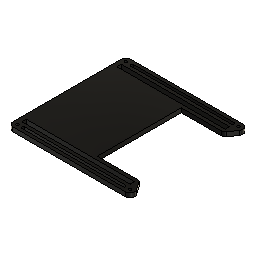
CameraBase v3 (Autodesk Fusion 360 design; units mm, degrees)
Autodesk Fusion 360 part; units mm, degrees
note: some values were not read from the file. Set by a fixed rule: which sketch regions a step uses.
sketch "Sketch1" plane through (0, 0, 0) normal (0, 0, 1) x (1, 0, 0)
  line L0 (-62.5, 60.2) -> (62.5, 60.2) construction
  line L1 (62.5, 60.2) -> (62.5, -60.2) construction
  line L2 (62.5, -60.2) -> (-62.5, -60.2) construction
  line L3 (-62.5, -60.2) -> (-62.5, 60.2) construction
  line L4 (0, 0) -> (0, 60.2) construction
  line L5 (0, 0) -> (-62.5, 0) construction
  circle A0 centre (62.5, 60.2) radius 1.5
  circle A1 centre (-62.5, 60.2) radius 1.5
  circle A2 centre (62.5, -60.2) radius 1.5
  circle A3 centre (-62.5, -60.2) radius 1.5
  line L6 (-62.5, -65.2) -> (62.5, -65.2)
  line L7 (-67.5, -60.2) -> (-67.5, 60.2)
  line L8 (-62.5, 65.2) -> (62.5, 65.2)
  line L9 (-56, 61.7) -> (56, 61.7)
  line L10 (-56, 58.7) -> (56, 58.7)
  arc A4 (-56, 61.7) -> (-56, 58.7) centre (-56, 60.2) ccw
  arc A5 (56, 58.7) -> (56, 61.7) centre (56, 60.2) ccw
  arc A6 (-67.5, 60.2) -> (-62.5, 65.2) centre (-62.5, 60.2) ccw construction
  arc A7 (-62.5, 65.2) -> (-67.5, 60.2) centre (-62.5, 60.2) ccw
  line L11 (-62.5, 55.2) -> (57.5, 55.2)
  line L12 (57.5, 55.2) -> (57.5, 50.4)
  line L13 (57.5, 50.4) -> (-62.5, 50.4)
  line L14 (-62.5, 50.4) -> (-62.5, 55.2)
  line L15 (66.6668, 57.4363) -> (60.6251, 48.3272)
  arc A8 (62.5, 65.2) -> (66.6668, 57.4363) centre (62.5, 60.2) ccw construction
  arc A9 (66.6668, 57.4363) -> (62.5, 65.2) centre (62.5, 60.2) ccw
  arc A10 (60.6251, 48.3272) -> (60.6251, 48.3272) centre (57.5, 50.4) ccw construction
  line L16 (-56, -58.7) -> (56, -58.7)
  line L17 (-56, -61.7) -> (56, -61.7)
  arc A11 (-56, -58.7) -> (-56, -61.7) centre (-56, -60.2) ccw
  arc A12 (56, -61.7) -> (56, -58.7) centre (56, -60.2) ccw
  line L18 (-62.5, -55.2) -> (57.5, -55.2)
  line L19 (57.5, -55.2) -> (57.5, -50.4)
  line L20 (57.5, -50.4) -> (-62.5, -50.4)
  line L21 (-62.5, -50.4) -> (-62.5, -55.2)
  line L22 (57.5, -60.2) -> (57.5, -55.2) construction
  line L23 (60.6251, -48.3272) -> (66.6668, -57.4363)
  line L24 (57.5, -46.65) -> (12.5, -46.65)
  line L25 (12.5, 46.65) -> (12.5, -46.65)
  arc A13 (57.5, -46.65) -> (60.6251, -48.3272) centre (57.5, -50.4) ccw construction
  arc A14 (60.6251, -48.3272) -> (57.5, -46.65) centre (57.5, -50.4) ccw
  arc A15 (66.6668, -57.4363) -> (62.5, -65.2) centre (62.5, -60.2) ccw construction
  arc A16 (62.5, -65.2) -> (66.6668, -57.4363) centre (62.5, -60.2) ccw
  arc A17 (-62.5, -65.2) -> (-67.5, -60.2) centre (-62.5, -60.2) ccw construction
  arc A18 (-67.5, -60.2) -> (-62.5, -65.2) centre (-62.5, -60.2) ccw
  line L26 (57.5, -50.4) -> (57.5, 50.4) construction
  line L27 (57.5, 46.65) -> (12.5, 46.65)
  arc A19 (60.6251, 48.3272) -> (57.5, 46.65) centre (57.5, 50.4) ccw construction
  arc A20 (57.5, 46.65) -> (60.6251, 48.3272) centre (57.5, 50.4) ccw
  line L28 (57.5, 55.2) -> (57.5, 60.2) construction
  point P0 (-62.5, 0)
  point P1 (0, 60.2)
  dimension "d1" = 125
  dimension "d2" = 120.4
  dimension "d3" = 3
  dimension "d4" = 3
  dimension "d5" = 3
  dimension "d6" = 3
  dimension "d7" = 10
  dimension "d8" = 10
  dimension "d9" = 10
  dimension "d10" = 10
  dimension "d11" = 3
  dimension "d12" = 5
  dimension "d13" = 6.5
  dimension "d14" = 6.5
  dimension "d16" = 4.8
  dimension "d17" = 5
  dimension "d19" = 3
  dimension "d20" = 5
  dimension "d21" = 6.5
  dimension "d22" = 6.5
  dimension "d23" = 4.8
  dimension "d24" = 7.5
  dimension "d25" = 50
  dimension "d28" = 3.75
  constraint horizontal L0
  constraint vertical L1
  constraint horizontal L2
  constraint vertical L3
  constraint midpoint L3 P0
  constraint midpoint L0 P1
  constraint coincident L4.start L5.start
  constraint coincident P1 L4.end
  constraint coincident P0 L5.end
  constraint vertical L4
  constraint horizontal L5
  constraint coincident L0.end L1.start
  constraint coincident L0.start L3.end
  constraint coincident L1.end L2.start
  constraint coincident L2.end L3.start
  constraint concentric A1 A6
  constraint concentric A0 A8
  constraint concentric A2 A15
  constraint concentric A3 A17
  constraint tangent L6 A15
  constraint perpendicular L1 L6
  constraint tangent L7 A6
  constraint perpendicular L6 L7
  constraint tangent L8 A8
  constraint perpendicular L7 L8
  constraint parallel L8 L9
  constraint parallel L0 L10
  constraint tangent L10 A4
  constraint tangent L9 A4
  constraint tangent L10 A5
  constraint tangent L9 A5
  constraint concentric A6 A7
  constraint horizontal L11
  constraint vertical L12
  constraint horizontal L13
  constraint vertical L14
  constraint coincident L3 L11.start
  constraint coincident L12.end L13.start
  constraint tangent L15 A10
  constraint tangent L15 A8
  constraint perpendicular L2 L25
  constraint concentric A8 A9
  constraint perpendicular L3 L16
  constraint parallel L16 L17
  constraint tangent L16 A11
  constraint tangent L17 A11
  constraint tangent L16 A12
  constraint tangent L17 A12
  constraint horizontal L18
  constraint vertical L19
  constraint horizontal L20
  constraint vertical L21
  constraint coincident L3 L18.start
  constraint midpoint A12 L22.start
  constraint tangent L22 A15
  constraint coincident L19.end L20.start
  constraint tangent L23 A15
  constraint tangent L23 A13
  constraint tangent L24 A13
  constraint perpendicular L24 L25
  constraint concentric A13 A14
  constraint concentric A15 A16
  constraint coincident L18.start A17
  constraint concentric A17 A18
  constraint vertical L26
  constraint coincident L26 L27.start
  constraint tangent A10 L27
  constraint tangent L15 A19
  constraint concentric A19 A20
  constraint collinear L12 L26
  constraint midpoint A5 L28.end
  constraint collinear L12 L28
  measures "d1" distance of L0.start L0.end
  measures "d2" distance of L0.start L2.end
  measures "d3" diameter of A0
  measures "d4" diameter of A1
  measures "d5" diameter of A2
  measures "d6" diameter of A3
  measures "d7" diameter of A6
  measures "d8" diameter of A8
  measures "d9" diameter of A15
  measures "d10" diameter of A17
  measures "d11" distance of L9 L10
  measures "d12" distance of L8 A4.centre
  measures "d13" distance of L0.start A4.centre
  measures "d14" distance of L0.end A5.centre
  measures "d16" distance of L11.start L13.end
  measures "d17" distance of L0 L11
  measures "d19" distance of L16 L17
  measures "d20" distance of L6 A11.centre
  measures "d21" distance of L2.end A11.centre
  measures "d22" distance of L1.end A12.centre
  measures "d23" distance of L18.start L20.end
  measures "d24" diameter of A13
  measures "d25" distance of L1 L25
  measures "d28" radius of A19
extrude "Extrude1" add sketch "Sketch1" along normal blind 4.8
